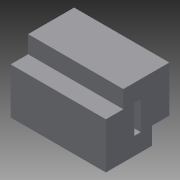
# Autodesk Inventor part: 148
Saved by Autodesk Inventor 2014 (Build 180170000, 170)
## iProperties
Created: 2017-04-22
Part Number: 148
Material: Generic
Document SubType Name: Modeling
Designer: Andy
Density: 1 g/cm^3
Appearance: Default
Author: Andy
Autodesk Inventor part; units mm, degrees
ref_plane "YZ Plane" through (0, 0, 0) normal (1, 0, 0) x (0, 1, 0)
ref_plane "XZ Plane" through (0, 0, 0) normal (0, 1, 0) x (-1, 0, 0)
ref_plane "XY Plane" through (0, 0, 0) normal (0, 0, 1) x (1, 0, 0)
sketch "Sketch1" plane through (0, 0, 0) normal (0, 1, 0) x (-1, 0, 0)
  line L0 (0, 0) -> (15, 0)
  line L1 (15, 0) -> (15, -10)
  line L2 (15, -10) -> (0, -10)
  line L3 (0, -10) -> (0, 0)
  dimension "d0" = 15
  dimension "d1" = 10
  constraints: 8 end point, 2 parallel, 1 horizontal, 1 perpendicular
  measures "d0" distance of L1.end L2.end
  measures "d1" distance of L0.end L1.end
extrude "Extrusion1" add sketch "Sketch1" along normal blind 10
sketch "Sketch2" plane through (-15, 0, 0) normal (0, 0, 1) x (1, 0, 0)
  line L0 (15, 0) -> (0, 0) projected
  line L1 (15, 0) -> (15, 10) projected
  line L2 (0, 0) -> (15, 0)
  line L3 (15, 0) -> (15, 2.75)
  line L4 (15, 2.75) -> (0, 2.75)
  line L5 (0, 2.75) -> (0, 0)
  dimension "d4" = 2.75
  constraints: 8 end point, 2 parallel, 1 horizontal, 1 perpendicular, 1 point on line
  measures "d4" distance of L3.end L2.end
extrude "Extrusion2" cut sketch "Sketch2" against normal blind 2.75
sketch "Sketch3" plane through (0, 0, -10) normal (1, 0, 0) x (0, 0, -1)
  line L0 (0, 10) -> (-2.75, 10)
  line L1 (-2.75, 10) -> (-2.75, 7.25)
  line L2 (-2.75, 7.25) -> (0, 7.25)
  line L3 (0, 7.25) -> (0, 10)
  point P0 (-10, 0)
  dimension "d7" = 2.75
  dimension "d8" = 2.75
  constraints: 8 end point, 2 parallel, 1 horizontal, 1 perpendicular
  measures "d7" distance of L2.end L1.end
  measures "d8" distance of L1.end L0.end
extrude "Extrusion3" cut sketch "Sketch3" against normal blind 15
sketch "Sketch4" plane through (0, 10, 0) normal (0, 1, 0) x (1, 0, 0)
  line L0 (0, 7.25) -> (-15, 7.25) projected
  line L1 (-10, 7.25) -> (-4, 7.25)
  line L2 (-4, 7.25) -> (-4, 4.5)
  line L3 (-4, 4.5) -> (-10, 4.5)
  line L4 (-10, 4.5) -> (-10, 7.25)
  dimension "d11" = 6
  dimension "d12" = 2.75
  constraints: 8 end point, 2 parallel, 1 horizontal, 1 perpendicular, 1 point on line
  measures "d11" distance of L2.end L3.end
  measures "d12" distance of L1.end L2.end
extrude "Extrusion4" cut sketch "Sketch4" against normal blind 2.75
sketch "Sketch5" plane through (0, 0, -2.75) normal (1, 0, 0) x (0, 0, -1)
  line L0 (0, 4.5) -> (4.5, 4.5)
  line L1 (4.5, 4.5) -> (4.5, 5.5)
  line L2 (4.5, 5.5) -> (0, 5.5)
  line L3 (0, 5.5) -> (0, 4.5)
  point P0 (-2.75, 0)
  dimension "d15" = 1
  constraints: 8 end point, 2 parallel, 1 horizontal, 1 perpendicular
  measures "d15" distance of L1.end L0.end
extrude "Extrusion5" cut sketch "Sketch5" against normal blind 15
body "Solid1"
